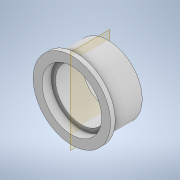
# Autodesk Inventor part: EDF Mount
Saved by Autodesk Inventor 2020 (Build 240168000, 168)
## iProperties
Created: 2020-03-02
Part Number: EDF Mount
Material: Generic
Document SubType Name: Modeling
Designer: pp445
Density: 1 g/cm^3
Appearance: Default
Author: pp445
Autodesk Inventor part; units mm, degrees
ref_plane "XZ Plane" through (0, 0, 0) normal (0, 1, 0) x (-1, 0, 0)
ref_plane "XY Plane" through (0, 0, 0) normal (0, 0, 1) x (1, 0, 0)
sketch "Sketch1" plane through (0, 0, 0) normal (0, 0, 1) x (1, 0, 0)
  circle A0 centre (0, 0) radius 27.575
  circle A1 centre (0, 0) radius 41.5
  dimension "d0" = 55.15
  dimension "d1" = 83
  constraints: 2 centre point, 2 coincident
  measures "d0" diameter of A0
  measures "d1" diameter of A1
extrude "Extrusion1" add sketch "Sketch1" along normal blind 39
sketch "Sketch2" plane through (0, 0, 0) normal (1, 0, 0) x (0, 1, 0)
  line L0 (41.5, 39) -> (-41.5, 39) projected
  line L1 (41.5, 0) -> (-41.5, 0) projected
  line L2 (42.7787, 29) -> (-54.5799, 29) construction
  line L3 (-27.575, 39) -> (27.575, 39) projected
  line L4 (-27.575, 39) -> (27.575, 39) projected
  line L5 (-27.575, 0) -> (27.575, 0) projected
  line L6 (41.5, 0) -> (27.575, 0) projected
  line L7 (27.575, 0) -> (27.575, 39) projected
  line L8 (27.575, 39) -> (41.5, 39) projected
  line L9 (-41.5, 39) -> (-27.575, 39) projected
  line L10 (-27.575, 39) -> (-27.575, 0) projected
  line L11 (-27.575, 0) -> (-41.5, 0) projected
  line L12 (27.575, 39) -> (32, 39)
  line L13 (32, 39) -> (32, 29)
  line L14 (32, 29) -> (27.575, 29)
  line L15 (27.575, 29) -> (27.575, 39)
  line L16 (0, -7.8) -> (0, 46.8) projected
  line L17 (41.5, 39) -> (41.5, 0) projected
  line L18 (-41.5, 0) -> (-41.5, 39) projected
  point P0 (0, 0)
  dimension "d4" = 10
  dimension "d5" = 32
  constraints: 10 end point, 3 parallel, 1 collinear, 1 horizontal, 1 perpendicular
  measures "d4" distance between parallel lines of L0 L2
  measures "d5" distance from line of point (0, 0) L13
revolve "Revolution1" cut sketch "Sketch2" angle 360 about axis through (0, 0, -10) along (0, 0, 1) contours L13 L14 L7 L0
sketch "Sketch3" plane through (0, 0, 0) normal (1, 0, 0) x (0, 1, 0)
  line L0 (41.5, 39) -> (41.5, 0) projected
  line L1 (41.5, 0) -> (27.575, 0) projected
  line L2 (27.575, 0) -> (27.575, 29) projected
  line L3 (27.575, 29) -> (32, 29) projected
  line L4 (32, 29) -> (32, 39) projected
  line L5 (32, 39) -> (41.5, 39) projected
  line L6 (-41.5, 0) -> (-41.5, 39) projected
  line L7 (-41.5, 39) -> (-32, 39) projected
  line L8 (-32, 39) -> (-32, 29) projected
  line L9 (-32, 29) -> (-27.575, 29) projected
  line L10 (-27.575, 29) -> (-27.575, 0) projected
  line L11 (-27.575, 0) -> (-41.5, 0) projected
  line L12 (-41.5, 0) -> (-41.5, 39) projected
  line L13 (-32, 39) -> (-32, 29) projected
  line L14 (-32, 34) -> (-41.5, 34)
  line L15 (-36.5, 34) -> (-36.5, 0)
  line L16 (41.5, 0) -> (-41.5, 0) projected
  line L17 (0, -7.8) -> (0, 46.8) projected
  point P0 (0, 0)
  dimension "d7" = 5
  dimension "d8" = 5
  constraints: 4 end point, 3 point on line, 1 midpoint, 1 parallel, 1 perpendicular
  measures "d7" distance between parallel lines of L7 L14
  measures "d8" distance between parallel lines of L6 L15
revolve "Revolution2" cut sketch "Sketch3" angle 360 about axis through (0, 0, -10) along (0, 0, 1) contours L6 L14 L15 L11
body "Solid1"
